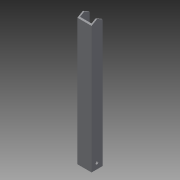
# Autodesk Inventor part: C-Channel - Cross Support
Saved by Autodesk Inventor 2013 (Build 170138000, 138)
## iProperties
Created: 2013-01-12
Part Number: C-Channel - Cross Support
Material: Generic
Document SubType Name: Modeling
Designer: carneeki
Density: 1 g/cm^3
Mass: 65.6443 g
Surface Area: 460.851 cm^2
Volume: 65.6443 cm^3
Author: carneeki
Autodesk Inventor part; units mm, degrees
ref_plane "YZ Plane" through (0, 0, 0) normal (1, 0, 0) x (0, 1, 0)
ref_plane "XZ Plane" through (0, 0, 0) normal (0, 1, 0) x (-1, 0, 0)
ref_plane "XY Plane" through (0, 0, 0) normal (0, 0, 1) x (1, 0, 0)
sketch "Sketch1" plane through (0, 0, 0) normal (0, 0, 1) x (1, 0, 0)
  line L0 (-16, -12.5) -> (16, -12.5)
  line L1 (16, -12.5) -> (16, 12.5)
  line L2 (16, 12.5) -> (13, 12.5)
  line L3 (13, 12.5) -> (13, -9.5)
  line L4 (13, -9.5) -> (-13, -9.5)
  line L5 (-13, -9.5) -> (-13, 12.5)
  line L6 (-13, 12.5) -> (-16, 12.5)
  line L7 (-16, 12.5) -> (-16, -12.5)
  point P0 (0, 0)
  dimension "d0" = 32
  dimension "d1" = 25
  dimension "d2" = 3
  dimension "d3" = 90
  dimension "d4" = 22
  dimension "d5" = 26
  dimension "d6" = 22
  dimension "d7" = 3
  dimension "d8" = 25
  dimension "d10" = 12.5
  dimension "d11" = 16
  constraints: 16 end point, 5 parallel, 1 horizontal, 1 perpendicular
  measures "d0" distance of L0.start L0.end
  measures "d1" distance of L0.end L1.end
  measures "d2" distance of L1.end L2.end
  measures "d3" angle of L2 L1
  measures "d4" distance of L2.end L3.end
  measures "d5" distance of L3.end L4.end
  measures "d6" distance of L4.end L5.end
  measures "d7" distance of L5.end L6.end
  measures "d8" distance of L6.end L0.start
  measures "d10" distance from line of point (0, 0) L2
  measures "d11" distance from line of point (0, 0) L1
extrude "Extrusion1" add sketch "Sketch1" against normal blind 293.2938
sketch "Sketch5" plane through (16, -12.5, 0) normal (1, 0, 0) x (0, 0, -1)
  line L0 (293.2938, 25) -> (293.2938, 0) projected
  line L1 (0, 25) -> (293.2938, 25) projected
  circle A0 centre (280.7938, 12.5) radius 3.175
  point P0 (0, 12.5)
  dimension "d51" = 25
  dimension "d52" = 6.35
  dimension "d53" = 12.5
  dimension "d54" = 12.5
  constraints: 1 centre point
  measures "d51" distance of L0.start L0.end
  measures "d52" diameter of A0
  measures "d53" distance from line of L1 A0.centre
  measures "d54" distance from line of A0.centre L0
hole "Hole2" at (16, 0, -280.7938) direction (-1, 0, 0) diameter 6.35 end through all
chamfer "Chamfer9" distance 12.5 angle 30 3 edges at (0, -12.5, 0) (-14.5, 12.5, 0) (14.5, 12.5, 0) measured on face at (-14.5, 12, 0) measured on face at (14.5, 12, 0) measured on face at (0, -12, 0)
equation "\"d5\" = d0 - 2 * d7"
equation "\"d10\" = 0.5 * d1"
equation "\"d11\" = 0.5 * d0"
equation "\"d53\" = 0.5 * d51"
equation "\"d54\" = d53"
body "Solid1"
